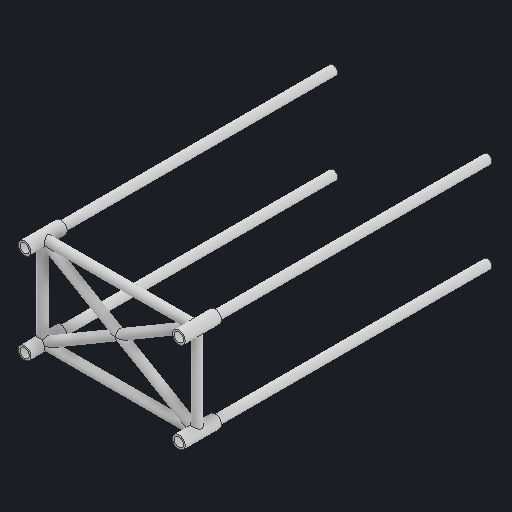
# Autodesk Inventor part: RCPlaneSkeletonMiddleFront2
Saved by Autodesk Inventor 2026.1 (Build 301233000, 233)
## iProperties
Created: 2026-03-11
Part Number: RCPlaneSkeletonMiddleFront2
Material: Generic
Document SubType Name: Modeling
Designer: morri
Density: 1 g/cm^3
Appearance: Default
Author: morri
Autodesk Inventor part; units mm, degrees
ref_plane "YZ Plane" through (0, 0, 0) normal (1, 0, 0) x (0, 1, 0)
sketch3d "3D Sketch1"
sketch "Sketch1" plane through (0, 0, 0) normal (0, 0, 1) x (1, 0, 0)
  line L0 (0, 0) -> (85, 0) construction
  line L1 (85, 0) -> (85, 50) construction
  line L2 (85, 50) -> (0, 50) construction
  line L3 (0, 50) -> (0, 0) construction
  circle A0 centre (0, 0) radius 2.5
  circle A1 centre (0, 50) radius 2.5
  circle A2 centre (85, 50) radius 2.5
  circle A3 centre (85, 0) radius 2.5
  dimension "d8" = 85
  dimension "d9" = 50
  dimension "d10" = 5
  dimension "d11" = 5
  dimension "d12" = 5
  dimension "d13" = 5
  constraints: 8 end point, 4 centre point, 4 coincident, 2 parallel, 1 horizontal, 1 perpendicular
  measures "d8" distance of L2.end L1.end
  measures "d9" distance of L1.end L0.end
  measures "d10" diameter of A0
  measures "d11" diameter of A1
  measures "d12" diameter of A2
  measures "d13" diameter of A3
extrude "Extrusion1" add sketch "Sketch1" against normal blind 150
sketch "Sketch2" plane through (0, 0, 0) normal (0, 0, 1) x (1, 0, 0)
  circle A0 centre (0, 0) radius 2.5 construction
  line L0 (0, 0) -> (85, 0) construction
  line L1 (85, 0) -> (85, 50) construction
  line L2 (85, 50) -> (0, 50) construction
  line L3 (0, 50) -> (0, 0) construction
  circle A1 centre (0, 0) radius 3.5
  circle A2 centre (0, 50) radius 2.5 projected
  circle A3 centre (0, 50) radius 3.5
  circle A4 centre (85, 50) radius 3.5
  circle A5 centre (85, 0) radius 3.5
  dimension "d16" = 85
  dimension "d17" = 50
  dimension "d18" = 7
  dimension "d19" = 7
  dimension "d20" = 7
  dimension "d21" = 7
  constraints: 8 end point, 4 centre point, 4 coincident, 2 parallel, 1 horizontal, 1 perpendicular
  measures "d16" distance of L2.end L1.end
  measures "d17" distance of L1.end L0.end
  measures "d18" diameter of A1
  measures "d19" diameter of A3
  measures "d20" diameter of A4
  measures "d21" diameter of A5
extrude "Extrusion2" add sketch "Sketch2" along normal blind 20 contours A1 | A2 | A3 | A4 | A5
sketch "Sketch3" plane through (0, 0, 20) normal (0, 0, 1) x (1, 0, 0)
  line L0 (0, 0) -> (85, 0) construction
  line L1 (85, 0) -> (85, 50) construction
  line L2 (85, 50) -> (0, 50) construction
  line L3 (0, 50) -> (0, 0) construction
  dimension "d24" = 85
  dimension "d25" = 50
  constraints: 8 end point, 2 parallel, 1 horizontal, 1 perpendicular
  measures "d24" distance of L2.end L1.end
  measures "d25" distance of L1.end L0.end
sketch "Sketch4" plane through (0, 0, 0) normal (1, 0, 0) x (0, 1, 0)
  line L0 (0, 0) -> (0, 10) construction
  circle A0 centre (0, 10) radius 2.5
  line L1 (0, 10) -> (50, 10) construction
  circle A1 centre (50, 10) radius 2.5
  dimension "d27" = 5
  dimension "d28" = 50
  dimension "d29" = 5
  constraints: 4 end point, 2 centre point, 2 coincident, 1 horizontal, 1 vertical
  measures "d27" diameter of A0
  measures "d28" distance of L1.start L1.end
  measures "d29" diameter of A1
extrude "Extrusion3" add sketch "Sketch4" along normal blind 85
sketch "Sketch5" plane through (0, 0, 0) normal (0, 1, 0) x (-1, 0, 0)
  line L0 (0, 0) -> (0, 10) construction
  line L1 (0, 10) -> (-85, 10) construction
  circle A0 centre (0, 10) radius 2.5
  circle A1 centre (-85, 10) radius 2.5
  dimension "d32" = 10
  dimension "d33" = 85
  dimension "d34" = 5
  dimension "d35" = 5
  constraints: 4 end point, 2 centre point, 2 coincident, 1 perpendicular, 1 vertical
  measures "d32" distance of L0.start L0.end
  measures "d33" distance of L0.end L1.end
  measures "d34" diameter of A0
  measures "d35" diameter of A1
extrude "Extrusion4" add sketch "Sketch5" along normal blind 50
ref_plane "Work Plane1" through (0, 0, 10) normal (0.8619, 0.507, 0) x (-0.507, 0.8619, 0)
ref_plane "Work Plane2" through (0, 50, 10) normal (0.8619, -0.507, 0) x (0.507, 0.8619, 0)
sketch "Sketch6" plane through (0, 0, 10) normal (0.8619, 0.507, 0) x (-0.507, 0.8619, 0)
  ellipse E0 centre (0, 0) end of major axis (0, 2.5) minor radius 0.8873 (-0.8784, 0.3536) -> (-0.8784, -0.3536) ccw construction
  circle A0 centre (0, 0) radius 2.5
  point P0 (0, -10)
  dimension "d42" = 5
  constraints: 1 centre point, 1 coincident, 1 other
  measures "d42" diameter of A0
sketch "Sketch7" plane through (0, 50, 10) normal (0.8619, -0.507, 0) x (0.507, 0.8619, 0)
  ellipse E0 centre (0, 0) end of major axis (0, 2.5) minor radius 0.8873 (-0.8784, 0.3536) -> (-0.8784, -0.3536) ccw construction
  circle A0 centre (0, 0) radius 2.5
  point P0 (-43.0967, -10)
  dimension "d43" = 5
  constraints: 1 centre point, 1 coincident, 1 other
  measures "d43" diameter of A0
sketch3d "3D Sketch2"
  line L0 (0, 0, 10) -> (85, 50, 10)
  dimension "d38" = 10
  dimension "d39" = 85
  dimension "d40" = 50
  dimension "d41" = 85
sweep "Sweep1" add profiles "Sketch6" path "3D Sketch2"
sketch3d "3D Sketch2 for Sweep2"
  line L0 (0, 50, 10) -> (85, 0, 10)
  dimension "d38" = 10
  dimension "d39" = 85
  dimension "d40" = 50
  dimension "d41" = 85
sweep "Sweep2" add profiles "Sketch7" path "3D Sketch2 for Sweep2"
hole "Hole1" at (0, 50, 20) at (85, 50, 20) at (85, 0, 20) at (0, 0, 20) direction (0, 0, -1) diameter 5.1 depth 15
equation "\"fitTol\" = 0.1"
body "Solid1"
